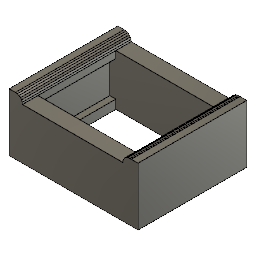
GPS-Wifi Case (Autodesk Fusion 360 archive; units mm, degrees)
design "Keystone Mount - Redesigned"
Autodesk Fusion 360 part; units mm, degrees
sketch "keystone-side" plane through (0, 0, 0) normal (0, 0, 1) x (1, 0, 0)
  line L0 (0.3425, -57.6967) -> (0.6681, -57.5618)
  line L1 (-19.7725, -68.7658) -> (-19.7725, -67.0158)
  line L2 (1.2775, -57.55) -> (1.2775, -57.5158)
  line L3 (-19.7725, -58.8658) -> (-0.3325, -58.8658)
  line L4 (-0.4364, -67.1264) -> (-3.5225, -68.7192)
  line L5 (2.6275, -57.5158) -> (2.6275, -68.7658)
  line L6 (1.0175, -57.5158) -> (1.2775, -57.55)
  line L7 (-3.5225, -68.7658) -> (-19.7725, -68.7658)
  line L8 (0.6681, -57.5618) -> (1.0175, -57.5158)
  line L9 (-20.9425, -67.0158) -> (-20.9425, -60.2158)
  line L10 (1.2775, -57.5158) -> (2.6275, -57.5158)
  line L11 (-19.9533, -58.1908) -> (-19.8185, -58.5164)
  line L12 (-19.7725, -58.8658) -> (-0.3325, -58.8658)
  line L13 (-20.9425, -60.2158) -> (-19.7725, -60.2158)
  line L14 (0.0629, -57.9112) -> (0.3425, -57.6967)
  line L15 (-0.3325, -58.8658) -> (-0.3325, -60.2158)
  line L16 (-0.1516, -58.1908) -> (0.0629, -57.9112)
  line L17 (-19.7725, -67.0158) -> (-20.9425, -67.0158)
  line L18 (2.6275, -68.7658) -> (-22.3725, -68.7658)
  line L19 (-20.7731, -57.5618) -> (-20.4475, -57.6967)
  line L20 (-0.3325, -60.2158) -> (1.1975, -60.2158)
  line L21 (-20.4475, -57.6967) -> (-20.1679, -57.9112)
  line L22 (-19.7725, -60.2158) -> (-19.7725, -58.8658)
  line L23 (1.1975, -67.0158) -> (-0.4934, -67.0158)
  line L24 (-22.3725, -57.5158) -> (-21.1225, -57.5158)
  line L25 (-22.3725, -68.7658) -> (-22.3725, -57.5158)
  line L26 (-21.1225, -57.5158) -> (-20.7731, -57.5618)
  line L27 (-0.4934, -67.0158) -> (-0.4364, -67.1264)
  line L28 (-20.1679, -57.9112) -> (-19.9533, -58.1908)
  line L29 (-19.8185, -58.5164) -> (-19.7725, -58.8658)
  line L30 (-0.2865, -58.5164) -> (-0.1516, -58.1908)
  line L31 (-3.5225, -68.7192) -> (-3.5225, -68.7658)
  line L32 (-0.3325, -58.8658) -> (-0.2865, -58.5164)
  line L33 (1.1975, -60.2158) -> (1.1975, -67.0158)
  line L34 (-19.7725, -60.2158) -> (-0.3325, -60.2158)
  constraint perpendicular L15 L34
extrude "Extrude1" add sketch "keystone-side" along normal blind 3
extrude "Extrude2" add sketch "keystone-side" against normal blind 18.1
extrude "Extrude3" cut sketch "keystone-side" against normal blind 15.1 contours L3 L12 L15 L22 L34 | L1 L4 L7 L9 L13 L17 L18 L20 L23 L27 L31 L33 L34
